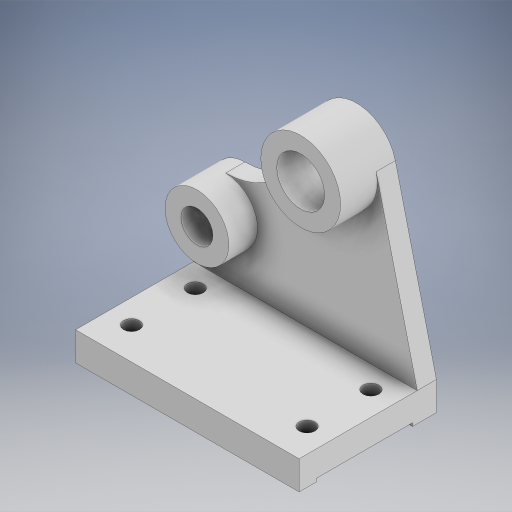
# Autodesk Inventor part: CE-1.3.4
Saved by Autodesk Inventor 2024 (Build 280153000, 153)
## iProperties
Created: 2024-01-25
Part Number: CE-1.3.4
Material: Generic
Document SubType Name: Modeling
Designer: Alex
Density: 1 g/cm^3
Appearance: Default
Author: Alex
Autodesk Inventor part; units mm, degrees
ref_plane "YZ Plane" through (0, 0, 0) normal (1, 0, 0) x (0, 1, 0)
ref_plane "XZ Plane" through (0, 0, 0) normal (0, 1, 0) x (-1, 0, 0)
sketch "Sketch1" plane through (0, 0, 0) normal (0, 1, 0) x (-1, 0, 0)
  line L0 (0, 0) -> (-140, 0)
  line L1 (-140, 0) -> (-140, -86)
  line L2 (-140, -86) -> (0, -86)
  line L3 (0, -86) -> (0, 0)
  line L4 (0, 0) -> (-15, 0) construction
  line L5 (-15, 0) -> (-15, -20) construction
  line L6 (-15, -20) -> (0, -20) construction
  line L7 (0, -20) -> (0, 0) construction
  circle A0 centre (-15, -20) radius 5
  line L8 (0, -43) -> (-140, -43) construction
  line L9 (-15, -20) -> (-125, -20) construction
  line L10 (-125, -20) -> (-125, -60) construction
  line L11 (-125, -60) -> (-15, -60) construction
  line L12 (-15, -60) -> (-15, -20) construction
  circle A1 centre (-125, -20) radius 5
  circle A2 centre (-125, -60) radius 5
  circle A3 centre (-15, -60) radius 5
  dimension "d0" = 140
  dimension "d1" = 86
  dimension "d2" = 15
  dimension "d3" = 20
  dimension "d4" = 10
  dimension "d5" = 110
  dimension "d6" = 40
  dimension "d7" = 10
  dimension "d8" = 10
  dimension "d9" = 10
  constraints: 26 end point, 6 parallel, 4 centre point, 4 coincident, 3 horizontal, 3 perpendicular, 2 midpoint
  measures "d0" distance of L2.end L1.end
  measures "d1" distance of L1.end L0.end
  measures "d2" distance of L6.end L5.end
  measures "d3" distance of L5.end L4.end
  measures "d4" diameter of A0
  measures "d5" distance of L11.end L10.end
  measures "d6" distance of L10.end L9.end
  measures "d7" diameter of A1
  measures "d8" diameter of A2
  measures "d9" diameter of A3
extrude "Extrusion1" add sketch "Sketch1" along normal blind 18
sketch "Sketch2" plane through (140, 0, 0) normal (1, 0, 0) x (0, 0, -1)
  line L0 (0, 18) -> (86, 18) construction
  line L1 (0, 0) -> (86, 0) construction
  line L2 (0, 18) -> (86, 18) construction
  line L3 (86, 18) -> (86, 0) construction
  line L4 (86, 0) -> (0, 0) construction
  line L5 (0, 0) -> (0, 18) construction
  line L6 (86, 0) -> (71, 0) construction
  line L7 (71, 0) -> (71, 2) construction
  line L8 (71, 2) -> (86, 2) construction
  line L9 (86, 2) -> (86, 0) construction
  line L10 (71, 2) -> (11, 2)
  line L11 (11, 2) -> (11, 0)
  line L12 (11, 0) -> (71, 0)
  line L13 (71, 0) -> (71, 2)
  dimension "d12" = 15
  dimension "d13" = 2
  dimension "d14" = 60
  constraints: 24 end point, 6 parallel, 3 horizontal, 3 perpendicular, 1 point on line
  measures "d12" distance of L7.end L8.end
  measures "d13" distance of L6.end L7.end
  measures "d14" distance of L12.end L11.end
extrude "Extrusion2" cut sketch "Sketch2" against normal up to surface (140 mm away)
ref_plane "Work Plane1" through (140, 9, -86) normal (0, 0, -1) x (-1, 0, 0)
sketch "Sketch3" plane through (140, 9, -86) normal (0, 0, -1) x (-1, 0, 0)
  line L0 (140, 9) -> (0, 9) construction
  line L1 (140, -9) -> (0, -9) construction
  line L2 (0, -9) -> (0, 9) construction
  line L3 (140, 9) -> (0, 9) projected
  line L4 (140, -9) -> (140, 9) construction
  line L5 (140, -9) -> (140, 9) construction
  circle A0 centre (120, 47) radius 20
  arc A1 (74.976, 110.0944) -> (120, 67) centre (120, 112.0672) ccw
  circle A2 centre (120, 47) radius 10
  line L6 (0, -9) -> (50, -9) construction
  line L7 (50, -9) -> (50, 109) construction
  line L8 (50, 109) -> (0, 109) construction
  line L9 (0, 109) -> (0, -9) construction
  circle A3 centre (50, 109) radius 25
  circle A4 centre (50, 109) radius 15
  line L10 (120, 47) -> (120, 67) construction
  line L11 (0, 9) -> (25.7055, 114.8972)
  line L12 (140, 9) -> (140, 47)
  dimension "d17" = 56
  dimension "d18" = 40
  dimension "d19" = 20
  dimension "d20" = 50
  dimension "d21" = 118
  dimension "d22" = 50
  dimension "d23" = 30
  constraints: 17 end point, 7 point on circle, 5 centre point, 5 tangent, 3 coincident, 3 vertical, 2 parallel, 1 horizontal, 1 perpendicular, 1 point on line
  measures "d17" distance of L1.start L12.end
  measures "d18" diameter of A0
  measures "d19" diameter of A2
  measures "d20" distance of L8.end L7.end
  measures "d21" distance of L7.end L6.end
  measures "d22" diameter of A3
  measures "d23" diameter of A4
extrude "Extrusion3" add sketch "Sketch3" against normal blind 12 contours L3 L11 A3 A1 A0 L12
extrude "Extrusion4" add sketch "Sketch3" against normal blind 35 contours A3
extrude "Extrusion5" add sketch "Sketch3" against normal blind 30 contours A0
body "Solid1"
